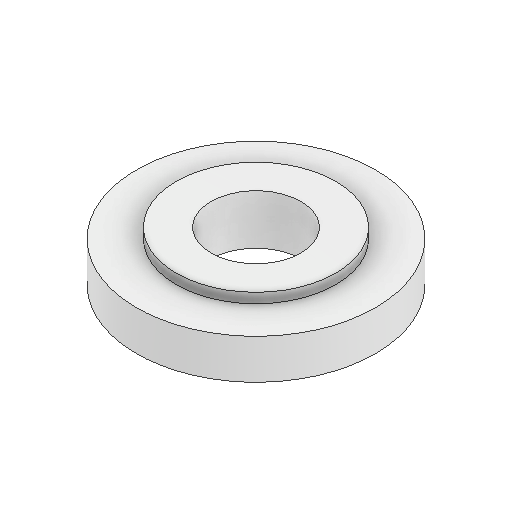
# Autodesk Inventor part: PivotWasher
Saved by Autodesk Inventor 2026.2 (Build 302298000, 298)
## iProperties
Created: 2026-03-24
Part Number: PivotWasher
Material: ABS Plastic
Document SubType Name: Modeling
Designer: gaoet
Density: 1.06 g/cm^3
Appearance: Smooth - White
Author: gaoet
Autodesk Inventor part; units mm, degrees
ref_plane "YZ Plane" through (0, 0, 0) normal (1, 0, 0) x (0, 1, 0)
ref_plane "XZ Plane" through (0, 0, 0) normal (0, 1, 0) x (-1, 0, 0)
ref_plane "XY Plane" through (0, 0, 0) normal (0, 0, 1) x (1, 0, 0)
sketch "Sketch1" plane through (0, 0, 0) normal (0, 0, 1) x (1, 0, 0)
  line L0 (0, 0) -> (0, 4.5652) construction
  line L1 (2.25, 0) -> (2.25, 2.5)
  line L2 (2.25, 2.5) -> (4, 2.5)
  line L3 (4, 2.5) -> (4, 2)
  line L4 (4, 2) -> (6, 2)
  line L5 (6, 2) -> (6, 0)
  line L6 (6, 0) -> (2.25, 0)
  point P0 (4, 2.25)
  dimension "d0" = 2.25
  dimension "d1" = 4
  dimension "d2" = 0.5
  dimension "d3" = 6
  dimension "d4" = 2
  constraints: 14 end point, 5 perpendicular, 2 vertical, 1 horizontal alignment, 1 midpoint
  measures "d0" distance between parallel lines of L0 L1
  measures "d1" distance from line of L0 point (4, 2.25)
  measures "d2" distance of L2.end L3.end
  measures "d3" distance between parallel lines of L0 L5
  measures "d4" distance of L4.end L5.end
revolve "Revolution1" add sketch "Sketch1" angle 360 about axis through (0, 0, 0) along (0, 1, 0)
body "Solid1"
